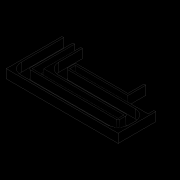
# Autodesk Inventor part: midPath
Saved by Autodesk Inventor 2022 (Build 260153000, 153)
## iProperties
Created: 2022-07-08
Part Number: midPath
Material: Generic
Document SubType Name: Modeling
Designer: Fuzzyfish
Density: 1 g/cm^3
Appearance: Default
Author: Fuzzyfish
Autodesk Inventor part; units mm, degrees
ref_plane "YZ Plane" through (0, 0, 0) normal (1, 0, 0) x (0, 1, 0)
ref_plane "XZ Plane" through (0, 0, 0) normal (0, 1, 0) x (-1, 0, 0)
ref_plane "XY Plane" through (0, 0, 0) normal (0, 0, 1) x (1, 0, 0)
sketch "Sketch1" plane through (0, 0, 0) normal (0, 1, 0) x (-1, 0, 0)
  line L0 (81.3062, -31.7218) -> (303.4779, -31.7218) construction
  line L1 (303.4779, -31.7218) -> (303.4779, -151.7218)
  line L2 (303.4779, -151.7218) -> (81.3062, -151.7218)
  line L3 (65.9779, -116.7218) -> (242.9779, -116.7218)
  line L4 (69.9779, -112.7218) -> (238.9779, -112.7218)
  line L5 (242.9779, -116.7218) -> (242.9779, -96.2218)
  line L6 (242.9779, -96.2218) -> (65.9779, -96.2218)
  line L7 (65.9779, -100.2218) -> (238.9779, -100.2218)
  line L8 (238.9779, -100.2218) -> (238.9779, -112.7218)
  arc A0 (242.9779, -100.2218) -> (238.9779, -96.2218) centre (238.9779, -100.2218) ccw
  arc A1 (238.9779, -116.7218) -> (242.9779, -112.7218) centre (238.9779, -112.7218) ccw
  line L9 (262.9779, -76.2218) -> (89.9779, -76.2218)
  line L10 (89.9779, -76.2218) -> (89.9779, -72.2218)
  line L11 (89.9779, -72.2218) -> (262.9779, -72.2218)
  line L12 (262.9779, -59.7218) -> (262.9779, -151.7218)
  line L13 (262.9779, -72.2218) -> (262.9779, -151.7218)
  line L14 (262.9779, -151.7218) -> (266.9779, -151.7218)
  line L15 (266.9779, -151.7218) -> (266.9779, -59.7218)
  line L16 (266.9779, -72.2218) -> (262.9779, -72.2218)
  line L17 (65.9779, -31.7218) -> (65.9779, -35.7218)
  line L18 (65.9779, -35.7218) -> (303.4779, -35.7218)
  line L19 (303.4779, -35.7218) -> (303.4779, -31.7218)
  line L20 (303.4779, -31.7218) -> (65.9779, -31.7218)
  line L21 (89.9779, -55.7218) -> (266.9779, -55.7218)
  line L22 (266.9779, -55.7218) -> (266.9779, -59.7218)
  line L23 (279.4779, -59.7218) -> (89.9779, -59.7218)
  line L24 (89.9779, -59.7218) -> (89.9779, -55.7218)
  line L25 (89.9779, -55.7218) -> (89.9779, -76.2218)
  line L26 (81.3062, -151.7218) -> (129.9779, -151.7218)
  line L27 (69.9779, -31.7218) -> (65.9779, -31.7218)
  line L28 (303.4779, -31.7218) -> (303.4779, -151.7218)
  line L29 (303.4779, -151.7218) -> (307.4779, -151.7218)
  line L30 (307.4779, -151.7218) -> (307.4779, -31.7218)
  line L31 (307.4779, -31.7218) -> (303.4779, -31.7218)
  line L32 (89.9779, -55.7218) -> (89.9779, -76.2218)
  line L33 (89.9779, -76.2218) -> (93.9779, -76.2218)
  line L34 (93.9779, -76.2218) -> (93.9779, -55.7218)
  line L35 (93.9779, -55.7218) -> (89.9779, -55.7218)
  line L36 (279.4779, -151.7218) -> (279.4779, -55.7218)
  line L37 (279.4779, -55.7218) -> (283.4779, -55.7218)
  line L38 (283.4779, -55.7218) -> (283.4779, -151.7218)
  line L39 (283.4779, -151.7218) -> (279.4779, -151.7218)
  line L40 (266.9779, -55.7218) -> (279.4779, -55.7218)
  line L41 (65.9779, -35.7218) -> (65.9779, -116.7218)
  line L42 (69.9779, -31.7218) -> (69.9779, -112.7218)
  line L43 (65.9779, -116.7218) -> (129.9779, -116.7218)
  line L44 (129.9779, -116.7218) -> (129.9779, -112.7218)
  line L45 (129.9779, -112.7218) -> (65.9779, -112.7218)
  line L46 (65.9779, -112.7218) -> (65.9779, -116.7218)
  line L47 (129.9779, -112.7218) -> (129.9779, -151.7218)
  line L48 (129.9779, -151.7218) -> (125.9779, -151.7218)
  line L49 (125.9779, -151.7218) -> (125.9779, -112.7218)
  line L50 (125.9779, -112.7218) -> (129.9779, -112.7218)
  point P0 (81.3062, -112.7218)
  point P1 (266.9779, -151.7218)
  point P2 (93.9779, -72.2218)
  point P3 (93.9779, -59.7218)
  point P4 (89.9779, -59.7218)
  point P5 (89.9779, -72.2218)
  point P6 (89.9779, -59.7218)
  point P7 (89.9779, -72.2218)
  point P8 (69.9779, -100.2218)
  point P9 (65.9779, -112.7218)
  point P10 (69.9779, -96.2218)
  point P11 (69.9779, -35.7218)
  dimension "d10" = 120
  dimension "d13" = 35
  dimension "d14" = 4
  dimension "d15" = 4
  dimension "d16" = 4
  dimension "d17" = 12.5
  dimension "d20" = 20
  dimension "d21" = 4
  dimension "d23" = 4
  dimension "d25" = 4
  dimension "d26" = 20
  dimension "d31" = 4
  dimension "d32" = 4
  dimension "d34" = 12.5
  dimension "d35" = 4
  dimension "d36" = 20
  dimension "d43" = 4
  dimension "d44" = 4
  dimension "d46" = 20
  dimension "d47" = 4
  dimension "d48" = 20
  dimension "d49" = 4
  dimension "d50" = 133
  dimension "d51" = 173
  constraints: 102 end point, 21 parallel, 19 point on line, 13 perpendicular, 7 horizontal, 7 vertical, 4 collinear, 4 point on circle, 2 centre point, 2 coincident
  measures "d10" distance of L2.end L0.start
  measures "d13" distance between parallel lines of L2 L3
  measures "d14" distance between parallel lines of L3 L4
  measures "d15" distance between parallel lines of L5 L8
  measures "d16" distance between parallel lines of L6 L7
  measures "d17" distance between parallel lines of L7 L4
  measures "d20" distance between parallel lines of L12 L5
  measures "d21" distance between parallel lines of L15 L13
  measures "d23" distance between parallel lines of L0 L18
  measures "d25" distance between parallel lines of L21 L23
  measures "d26" distance between parallel lines of L18 L21
  measures "d31" distance between parallel lines of L30 L1
  measures "d32" distance between parallel lines of L34 L32
  measures "d34" distance between parallel lines of L36 L15
  measures "d35" distance between parallel lines of L38 L36
  measures "d36" distance between parallel lines of L1 L38
  measures "d43" distance between parallel lines of L47 L49
  measures "d44" distance between parallel lines of L45 L43
  measures "d46" distance between parallel lines of L42 L25
  measures "d47" distance between parallel lines of L42 L41
  measures "d48" distance between parallel lines of L6 L9
  measures "d49" distance between parallel lines of L9 L11
  measures "d50" distance between parallel lines of L12 L47
  measures "d51" distance between parallel lines of L25 L12
extrude "Extrusion1" add sketch "Sketch1" along normal blind 19 contours L31 L30 L29 L1 | L1 L18 L42 L20 | L42 L18 L17 L20 | L42 L6 L41 L18 | L2 L36 L37 L38 | L42 L7 L41 L6 | L6 A0 L5 A1 L3 L44 L4 L8 L7 L42 | L42 L45 L41 L7 | L2 L12 L16 L15 | L23 L22 L40 L36 | L23 L34 L21 L22 | L4 L44 L3 L49 | L2 L49 L3 L47 | L9 L34 L11 L12 | L34 L23 L24 L21 | L9 L10 L11 L34 | L11 L25 L23 L34
fillet "Fillet1" radius 24 4 edges at (-303.4779, 9.5, -35.7218) (-262.9779, 9.5, -76.2218) (-69.9779, 9.5, -96.2218) (-69.9779, 9.5, -35.7218)
fillet "Fillet2" radius 4 3 edges at (-283.4779, 9.5, -55.7218) (-89.9779, 9.5, -55.7218) (-89.9779, 9.5, -76.2218)
body "Solid1"
